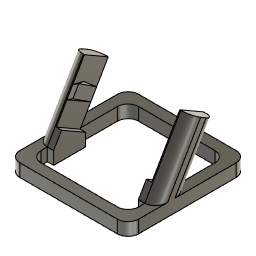
Hygrometer pedestal (Autodesk Fusion 360 design; units mm, degrees)
Autodesk Fusion 360 part; units mm, degrees
sketch "Sketch1" plane through (0, 0, 0) normal (0, 0, 1) x (1, 0, 0)
  line L0 (28, -28) -> (-28, -28)
  line L1 (-28, -28) -> (-28, 28)
  line L2 (-28, 28) -> (28, 28)
  line L3 (28, 28) -> (28, -28)
  line L4 (28, -28) -> (-28, 28) construction
  line L5 (-28, -28) -> (28, 28) construction
  dimension "d1" = 56
  dimension "d2" = 56
  constraint horizontal L0
  constraint perpendicular L0 L1
  constraint parallel L0 L2
  constraint parallel L1 L3
  constraint coincident L4 origin
  constraint coincident L5 origin
  measures "d1" distance of L1.end L2.end
  measures "d2" distance of L0.end L1.end
extrude "Extrude1" add sketch "Sketch1" along normal blind 6
sketch "Sketch2" plane through (28, 0, 0) normal (1, 0, 0) x (0, 1, 0)
  line L0 (-28, 0) -> (28, 0)
  line L1 (28, 0) -> (28, 6)
  line L2 (28, 6) -> (-28, 6)
  line L3 (-28, 6) -> (-28, 0)
  line L4 (-15.0687, 6) -> (1.934, 35.4497)
  line L5 (1.934, 35.4497) -> (13.1924, 28.9497)
  line L6 (13.1924, 28.9497) -> (-0.0576, 6)
  line L7 (7.5632, 32.1997) -> (-7.5632, 6) construction
  line L8 (0, 19.0998) -> (0, 6) construction
  dimension "d5" = 60
  dimension "d6" = 26.5
  dimension "d13" = 13
  constraint coincident L2 L4.start
  constraint perpendicular L4 L5
  constraint coincident L2 L6.end
  constraint perpendicular L5 L6
  constraint midpoint L5 L7.start
  constraint coincident L2 L7.end
  constraint perpendicular L5 L7
  constraint midpoint L7 L8.start
  constraint midpoint L2 L8.end
  constraint vertical L8
  measures "d5" angle of L2 L6
  measures "d6" distance of L5.end L6.end
  measures "d13" distance of L4.end L5.end
extrude "Extrude2" add sketch "Sketch2" against normal up to surface (56 mm away) contours L2 L4 L5 L6
sketch "Sketch3" plane through (0, -13.8996, 8.025) normal (0, -0.866025, 0.5) x (1, 0, 0)
  line L0 (-28, 31.6673) -> (-28, -2.3382)
  line L1 (-28, -2.3382) -> (28, -2.3382)
  line L2 (28, -2.3382) -> (28, 31.6673)
  line L3 (28, 31.6673) -> (-28, 31.6673)
  line L4 (22.5, 31.6673) -> (22.5, 5.1673)
  line L5 (22.5, 5.1673) -> (0, 5.1673)
  line L6 (0, 5.1673) -> (-22.5, 5.1673)
  line L7 (-22.5, 5.1673) -> (-22.5, 31.6673)
  line L8 (0, -2.3382) -> (0, 5.1673) construction
  dimension "d9" = 45
  dimension "d10" = 26.5
  constraint coincident L3 L4.start
  constraint perpendicular L3 L4
  constraint perpendicular L4 L5
  constraint perpendicular L4 L6
  constraint coincident L3 L7.end
  constraint perpendicular L3 L7
  constraint equal L5 L6
  constraint midpoint L1 L8.start
  constraint perpendicular L1 L8
  constraint coincident L5.end L6.start
  measures "d9" distance of L4 L7
  measures "d10" distance of L4.start L4.end
extrude "Extrude3" cut sketch "Sketch3" against normal up to surface (13 mm away) contours L3 L4 L5 L6 L7
sketch "Sketch4" plane through (0, 15.8337, 27.4247) normal (0, 0.5, 0.866025) x (-1, 0, 0)
  line L0 (22.5, 16.0499) -> (22.5, 3.0499)
  line L1 (22.5, 3.0499) -> (28, 3.0499)
  line L2 (28, 3.0499) -> (28, 16.0499)
  line L3 (28, 16.0499) -> (22.5, 16.0499)
  line L4 (22.5, 11.0499) -> (24, 11.0499) construction
  line L5 (24, 11.0499) -> (22.5, 3.0499)
  line L6 (24, 11.0499) -> (22.5, 16.0499)
  line L7 (-24, 11.0499) -> (-22.5, 16.0499)
  line L8 (-24, 11.0499) -> (-22.5, 3.0499)
  line L9 (-22.5, 3.0499) -> (-22.5, 16.0499)
  line L10 (-22.5, 11.0499) -> (-24, 11.0499) construction
  line L11 (22.5, 9.5499) -> (-22.5, 9.5499) construction
  line L12 (22.5, 11.0499) -> (-22.5, 11.0499) construction
  point P0 (-22.5, 16.0499)
  point P1 (-22.5, 3.0499)
  dimension "d27" = 48
  dimension "d29" = 1.5
  constraint perpendicular L0 L4
  constraint coincident L0.end L1.start
  constraint coincident L0.start L3.end
  constraint coincident P0 L7.end
  constraint coincident P1 L8.end
  constraint perpendicular L9 L10
  constraint equal L4 L10
  constraint coincident L9 L10.start
  constraint coincident L0 L4.start
  constraint midpoint L0 L11.start
  constraint midpoint L9 L11.end
  constraint parallel L11 L12
  measures "d27" distance of L4.end L7.start
  measures "d29" distance of L10.start L11
extrude "Extrude4" cut sketch "Sketch4" against normal up to surface (7 mm away) from surface at -9.5 contours L0 L5 L6 | L7 L8 L9
sketch "Sketch5" plane through (0, 0, 6) normal (0, 0, 1) x (-1, 0, 0)
  line L0 (28, -28) -> (28, 0.0576)
  line L1 (28, 0.0576) -> (22.5, 0.0576)
  line L2 (-28, 0.0576) -> (-28, -28)
  line L3 (-28, -28) -> (28, -28)
  line L4 (-23, 0.0576) -> (-23, -23)
  line L5 (-23, -23) -> (0, -23)
  line L6 (0, -23) -> (23, -23)
  line L7 (23, 0.0576) -> (23, -23)
  line L8 (0, 0) -> (0, -23) construction
  line L9 (-28, 15.0687) -> (28, 15.0687)
  line L10 (23, 0.0576) -> (23, 15.0687) construction
  line L11 (-23, 0.0576) -> (-23, 15.0687) construction
  line L12 (-23, 15.0687) -> (-23, 23)
  line L13 (-23, 23) -> (23, 23)
  line L14 (23, 15.0687) -> (23, 23)
  line L15 (-23, 23) -> (-23, 28) construction
  line L16 (28, 28) -> (-28, 28) construction
  line L17 (-23, -23) -> (-23, -28) construction
  line L18 (-23, -23) -> (-28, -23) construction
  line L19 (22.5, 0.0576) -> (-22.5, 0.0576)
  line L20 (-22.5, 0.0576) -> (-28, 0.0576)
  dimension "d24" = 5
  constraint coincident L1 L4.start
  constraint perpendicular L1 L4
  constraint perpendicular L4 L5
  constraint perpendicular L4 L6
  constraint coincident L1 L7.start
  constraint perpendicular L6 L7
  constraint equal L5 L6
  constraint coincident L8.start origin
  constraint vertical L8
  constraint coincident L9 L10.end
  constraint perpendicular L9 L10
  constraint coincident L9 L11.end
  constraint perpendicular L9 L11
  constraint perpendicular L9 L12
  constraint perpendicular L12 L13
  constraint perpendicular L13 L14
  constraint perpendicular L13 L15
  constraint coincident L15.end L16
  constraint perpendicular L5 L17
  constraint coincident L3 L17.end
  constraint perpendicular L17 L18
  constraint coincident L2 L18.end
  constraint equal L17 L18
  constraint equal L15 L18
  measures "d24" distance of L4.end L18.end
extrude "Extrude5" cut sketch "Sketch5" against normal through all contours L1 L4 L5 L6 L7 L19 L20 | L9 L12 L13 L14
fillet "Fillet1" radius 5 8 edges at (28, 28, 3) (-28, 28, 3) (28, -28, 3) (-28, -28, 3) (23, 23, 3) (-23, 23, 3) (23, -23, 3) (-23, -23, 3)
fillet "Fillet2" radius 5 4 edges at (28, -6.5674, 20.7248) (28, 6.5674, 17.4748) (-28, -6.5674, 20.7248) (-28, 6.5674, 17.4748)
sketch "Sketch6" plane through (0, 0, 0) normal (0, 0, -1) x (1, 0, 0)
  arc A0 (-23, 28) -> (-28, 23) centre (-23, 23) ccw
  line L0 (-28, 23) -> (-28, -23)
  arc A1 (-28, -23) -> (-23, -28) centre (-23, -23) ccw
  line L1 (-23, -28) -> (23, -28)
  arc A2 (23, -28) -> (28, -23) centre (23, -23) ccw
  line L2 (28, -23) -> (28, 23)
  arc A3 (28, 23) -> (23, 28) centre (23, 23) ccw
  line L3 (23, 28) -> (-23, 28)
  line L4 (-23, -18) -> (-23, 0.0576)
  line L5 (-23, 0.0576) -> (23, 0.0576)
  line L6 (23, 0.0576) -> (23, -18)
  arc A4 (18, -23) -> (23, -18) centre (18, -18) ccw
  line L7 (18, -23) -> (-18, -23)
  arc A5 (-23, -18) -> (-18, -23) centre (-18, -18) ccw
  line L8 (23, 18) -> (23, 15.0687)
  line L9 (23, 15.0687) -> (-23, 15.0687)
  line L10 (-23, 15.0687) -> (-23, 18)
  arc A6 (-18, 23) -> (-23, 18) centre (-18, 18) ccw
  line L11 (-18, 23) -> (18, 23)
  arc A7 (23, 18) -> (18, 23) centre (18, 18) ccw
  line L12 (-23, 0.0576) -> (23, 0.0576)
  line L13 (23, 15.0687) -> (-23, 15.0687)
  line L14 (20, 0.0576) -> (20, 15.0687)
  line L15 (-20, 15.0687) -> (-20, 0.0576)
  line L16 (20, 7.5632) -> (0, 7.5632) construction
  line L17 (0, 7.5632) -> (0, 0) construction
  line L18 (0, 7.5632) -> (-20, 7.5632) construction
  dimension "d25" = 3
  constraint coincident L12 L14.start
  constraint coincident L9 L14.end
  constraint perpendicular L9 L14
  constraint coincident L13 L15.start
  constraint coincident L12 L15.end
  constraint perpendicular L12 L15
  constraint midpoint L14 L16.start
  constraint perpendicular L14 L16
  constraint coincident L17.end origin
  constraint perpendicular L16 L17
  constraint midpoint L15 L18.end
  constraint equal L16 L18
  measures "d25" distance of L4.end L15.end
extrude "Extrude6" cut sketch "Sketch6" against normal through all contours L5 L9 L12 L13 L14 L15
chamfer "Chamfer1" distance 1.45 angle 45 4 edges at (23.25, 4.9783, 22.7224) (23.25, -0.6509, 25.9724) (-23.25, 4.9783, 22.7224) (-23.25, -0.6509, 25.9724)
